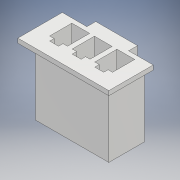
# Autodesk Inventor part: Connecteur JST 3 Broches Male
Saved by Autodesk Inventor 2017 (Build 210142000, 142)
## iProperties
Part Number: Connecteur JST 3 Broches Male
Material: Plastique ABS
Document SubType Name: Modeling
Designer: Adrien MARY
Mass: 0.175381 g
Surface Area: 5.51033 cm^2
Volume: 0.165454 cm^3
Density: 1.06 g/cm^3
Appearance: Lisse - Blanc
GlobalPropertyList: <PropertyList/>
Author: Adrien MARY
Autodesk Inventor part; units mm, degrees
ref_plane "YZ Plane" through (0, 0, 0) normal (1, 0, 0) x (0, 1, 0)
ref_plane "XZ Plane" through (0, 0, 0) normal (0, 1, 0) x (-1, 0, 0)
ref_plane "XY Plane" through (0, 0, 0) normal (0, 0, 1) x (1, 0, 0)
sketch "Esquisse1" plane through (0, 0, 0) normal (0, 0, 1) x (1, 0, 0)
  line L0 (-4.12, -2) -> (4.12, -2)
  line L1 (4.12, -2) -> (4.12, 2)
  line L2 (4.12, 2) -> (-4.12, 2)
  line L3 (-4.12, 2) -> (-4.12, -2)
  line L4 (-4.12, -2) -> (4.12, 2) construction
  line L5 (4.12, -2) -> (-4.12, 2) construction
  point P0 (0, 0)
  dimension "d0" = 8.24
  dimension "d1" = 4
  constraints: 12 end point, 2 midpoint, 2 parallel, 1 horizontal, 1 perpendicular
  measures "d0" distance of L2.end L1.end
  measures "d1" distance of L1.end L0.end
extrude "Embase" add sketch "Esquisse1" along normal blind 7.5
sketch "Esquisse2" plane through (0, 0, 7.5) normal (0, 0, 1) x (1, 0, 0)
  line L0 (-5.12, -3) -> (5.12, -3)
  line L1 (5.12, -3) -> (5.12, 2)
  line L2 (5.12, 2) -> (-5.12, 2)
  line L3 (-5.12, 2) -> (-5.12, -3)
  line L4 (-5.12, -3) -> (5.12, 2) construction
  line L5 (5.12, -3) -> (-5.12, 2) construction
  line L6 (4.12, 2) -> (-4.12, 2) projected
  line L7 (4.12, -2) -> (4.12, 2) projected
  point P0 (0, -0.5)
  point P1 (0, 0)
  point P2 (0, -0.5)
  dimension "d5" = 5
  dimension "d9" = 1
  constraints: 12 end point, 3 midpoint, 2 parallel, 1 collinear, 1 horizontal, 1 perpendicular, 1 vertical alignment
  measures "d5" distance of L1.end L0.end
  measures "d9" distance between parallel lines of L1 L7
extrude "Epaulement" add sketch "Esquisse2" along normal blind 0.5
sketch "Esquisse4" plane through (-4.12, 2, 0) normal (0, 1, 0) x (1, 0, 0)
  line L0 (5.87, -2) -> (5.87, -7.4)
  line L1 (5.87, -7.4) -> (2.37, -7.4)
  line L2 (2.37, -7.4) -> (2.37, -2)
  line L3 (2.37, -2) -> (1.87, -2)
  line L4 (1.87, -2) -> (1.12, -3)
  line L5 (1.12, -4) -> (1.77, -4)
  line L6 (1.77, -4) -> (1.77, -8)
  line L7 (1.77, -8) -> (6.47, -8)
  line L8 (6.47, -8) -> (6.47, -4)
  line L9 (6.47, -4) -> (7.12, -4)
  line L10 (7.12, -3) -> (6.37, -2)
  line L11 (6.37, -2) -> (5.87, -2)
  line L12 (8.24, 0) -> (0, 0) projected
  line L13 (9.24, -8) -> (-1, -8) construction
  line L14 (7.12, -3) -> (7.12, -4)
  line L15 (1.12, -4) -> (1.12, -3)
  point P0 (4.12, 0)
  point P1 (4.12, -7.4)
  point P2 (4.12, 0)
  dimension "d10" = 0.6
  dimension "d11" = 0.6
  dimension "Entre_clip" = 3.5
  dimension "d13" = 6
  dimension "d14" = 4
  dimension "d15" = 1
  dimension "d16" = 0.6
  dimension "d18" = 0.5
  dimension "d21" = 0.65
  constraints: 28 end point, 8 perpendicular, 3 equal length, 2 midpoint, 2 vertical, 1 collinear, 1 horizontal, 1 horizontal alignment, 1 parallel, 1 point on line, 1 vertical alignment
  measures "d10" distance between parallel lines of L8 L0
  measures "d11" distance between parallel lines of L7 L1
  measures "Entre_clip" distance between parallel lines of L2 L0
  measures "d13" distance between parallel lines of L7 L11
  measures "d14" distance between parallel lines of L13 L5
  measures "d15" distance of L10.start L9.end
  measures "d16" distance between parallel lines of L2 L6
  measures "d18" distance of L2.end L3.end
  measures "d21" distance of L5.start L5.end
extrude "Clip" add sketch "Esquisse4" along normal blind 1
sketch "Esquisse5" plane through (0, 0, 8) normal (0, 0, 1) x (1, 0, 0)
  line L0 (3.54, -1) -> (3.54, 1.5)
  line L1 (3.54, 1.5) -> (1.54, 1.5)
  line L2 (1.54, 1.5) -> (1.54, -1)
  line L3 (5.12, -3) -> (5.12, 2) projected
  line L4 (2.54, 1.25) -> (2.54, -1.75) construction
  line L5 (3.04, -1) -> (3.04, -1.4998)
  line L6 (3.04, -1.4998) -> (2.04, -1.4998)
  line L7 (2.04, -1.4998) -> (2.04, -1)
  line L8 (1.54, -1) -> (2.04, -1)
  line L9 (3.04, -1) -> (3.54, -1)
  line L10 (5.12, 2) -> (2.35, 2) projected
  point P0 (0, 0)
  point P1 (2.04, 1.5)
  point P2 (3.54, 0.25)
  point P3 (5.12, -0.5)
  point P4 (2.54, -1.713)
  point P5 (2.54, -1.4998)
  point P6 (2.54, 1.5)
  dimension "d22" = 2.58
  dimension "d24" = 2.5
  dimension "d34" = 0.4998
  dimension "d35" = 1
  dimension "d36" = 2
  dimension "d37" = 0.5
  constraints: 19 end point, 10 perpendicular, 4 midpoint, 3 vertical alignment, 1 collinear, 1 point on line, 1 vertical
  measures "d22" distance between parallel lines of L3 L4
  measures "d24" distance of L0.start L0.end
  measures "d34" distance of L6.end L7.end
  measures "d35" distance of L5.end L6.end
  measures "d36" distance between parallel lines of L0 L2
  measures "d37" distance between parallel lines of L10 L1
extrude "Extrusion4" cut sketch "Esquisse5" against normal blind 7
sketch "Esquisse6" plane through (0, 0, 1) normal (0, 0, 1) x (1, 0, 0)
  line L0 (2.04, 0) -> (3.04, 0)
  line L1 (3.04, 0) -> (3.04, 1)
  line L2 (3.04, 1) -> (2.04, 1)
  line L3 (2.04, 1) -> (2.04, 0)
  line L4 (2.04, -1) -> (1.54, -1) projected
  line L5 (1.54, 1.5) -> (3.54, 1.5) projected
  line L6 (3.04, -1.4998) -> (2.04, -1.4998) projected
  point P0 (0, 0)
  point P1 (2.54, 1)
  point P2 (2.96, -1.75)
  point P3 (2.54, 0)
  point P4 (2.54, -1.4998)
  dimension "d29" = 1
  dimension "d30" = 1
  dimension "d38" = 0.5
  constraints: 8 end point, 3 midpoint, 2 parallel, 1 horizontal, 1 perpendicular, 1 vertical alignment, 1 other
  measures "d29" distance of L0.end L1.end
  measures "d30" distance of L0.start L0.end
  measures "d38" distance between parallel lines of L5 L2
extrude "Extrusion5" cut sketch "Esquisse6" against normal through all
pattern_linear "Réseau rectangulaire1" count 3 spacing 2.54 along (-1, 0, 0) of "Extrusion4", "Extrusion5"
equation "\"d11\" = d10"
equation "\"Entre_clip\" = 1.16667 * Nb_broche"
equation "\"d16\" = d11"
equation "\"Pas\" = 2.54"
equation "\"Nb_broche\" = 3"
